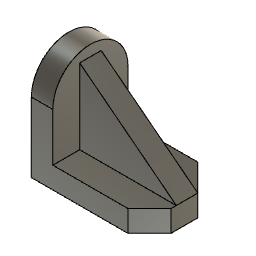
A1 (Autodesk Fusion 360 design; units mm, degrees)
Autodesk Fusion 360 part; units mm, degrees
sketch "Sketch1" plane through (0, 0, 0) normal (0, 0, 1) x (1, 0, 0)
  line L0 (51, 42) -> (0, 42)
  line L1 (0, 42) -> (0, 0)
  line L2 (0, 0) -> (54, 0)
  line L3 (54, 0) -> (66, 12)
  line L4 (66, 12) -> (66, 27)
  line L5 (66, 27) -> (51, 42)
  constraint horizontal L0
  constraint vertical L1
  constraint coincident L1.end L2.start
  constraint perpendicular L1 L2
  constraint perpendicular L0 L4
  constraint perpendicular L3 L5
extrude "Extrude1" add sketch "Sketch1" along normal blind 12 makes body 1
sketch "Sketch2" plane through (0, 0, 0) normal (0, 0, 1) x (1, 0, 0)
  line L0 (0, 0) -> (12, 0)
  line L1 (12, 0) -> (12, 42)
  line L2 (12, 42) -> (0, 42)
  line L3 (0, 42) -> (0, 0)
  constraint horizontal L0
  constraint vertical L1
  constraint horizontal L2
  constraint vertical L3
  constraint coincident L0.start L3.end
extrude "Extrude2" add sketch "Sketch2" along normal blind 39 bodies 1
sketch "Sketch3" plane through (0, 0, 0) normal (1, 0, 0) x (0, 1, 0)
  line L0 (42, 39) -> (0, 39)
  arc A0 (42, 39) -> (0, 39) centre (21, 39) ccw
  constraint horizontal L0
extrude "Extrude3" add sketch "Sketch3" along normal blind 12 bodies 1
sketch "Sketch4" plane through (0, 0, 0) normal (0, 1, 0) x (1, 0, 0)
  line L0 (12, -12) -> (12, -54)
  line L1 (12, -54) -> (66, -12)
  line L2 (66, -12) -> (12, -12)
  constraint vertical L0
  constraint perpendicular L0 L2
extrude "Extrude4" add sketch "Sketch4" along normal blind 12 separate body makes body 2
move_body "Move1" bodies 2 to x (1, 0, 0) y (0, 1, 0) z (0, 0, 1) at (0, 15, 0)
combine "Combine1" operation add target body 1 tool bodies 2
named bodies: "A1"
